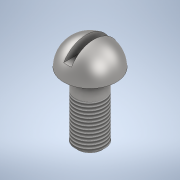
# Autodesk Inventor part: Parafuso
Saved by Autodesk Inventor 2021 (Build 250183000, 183)
## iProperties
Created: 2021-04-08
Part Number: Parafuso
Material: Genérico
Document SubType Name: Modeling
Designer: rubia
Density: 1 g/cm^3
Appearance: Inoxidável - Escovado
Author: rubia
Autodesk Inventor part; units mm, degrees
ref_plane "YZ Plane" through (0, 0, 0) normal (1, 0, 0) x (0, 1, 0)
ref_plane "XY Plane" through (0, 0, 0) normal (0, 0, 1) x (1, 0, 0)
sketch "Esboço1" plane through (0, 0, 0) normal (0, 0, 1) x (1, 0, 0)
  line L0 (-2.25, 0) -> (-2.25, -10)
  line L1 (-2.25, -10) -> (0, -10)
  line L2 (0, -10) -> (0, 0)
  line L3 (0, 0) -> (0, 4)
  line L4 (-2.25, 0) -> (-4, 0)
  arc A0 (0, 4) -> (-4, 0) centre (0, 0) ccw
  dimension "d1" = 2.25
  dimension "d2" = 10
  constraints: 10 end point, 2 point on circle, 1 centre point, 1 coincident, 1 parallel, 1 perpendicular, 1 vertical
  measures "d1" distance of L1.end L0.end
  measures "d2" distance of L0.end L0.start
revolve "Revolução1" add sketch "Esboço1" angle 360 about axis through (0, -10, 0) along (0, 1, 0)
thread "Rosca1" size "M4.5x0.5" class "6g" standard "ANSI Metric M Profile" length 7
chamfer "Chanfro1" distance 0.4 angle 45 1 edges at (2.25, -10, 0)
ref_plane "Plano de trabalho1" through (0, 4, 0) normal (0, 1, 0) x (-1, 0, 0)
sketch "Esboço2" plane through (0, 4, 0) normal (0, 1, 0) x (-1, 0, 0)
  line L0 (0.6, -6.0887) -> (-0.6, -6.0887)
  line L1 (-0.6, -6.0887) -> (-0.6, 6.0887)
  line L2 (-0.6, 6.0887) -> (0.6, 6.0887)
  line L3 (0.6, 6.0887) -> (0.6, -6.0887)
  line L4 (0.6, -6.0887) -> (-0.6, 6.0887) construction
  line L5 (-0.6, -6.0887) -> (0.6, 6.0887) construction
  point P0 (0, 0)
  dimension "d10" = 1.2
  constraints: 12 end point, 2 midpoint, 2 parallel, 1 horizontal, 1 perpendicular
  measures "d10" distance of L1.end L2.end
extrude "Extrusão1" cut sketch "Esboço2" against normal blind 2
